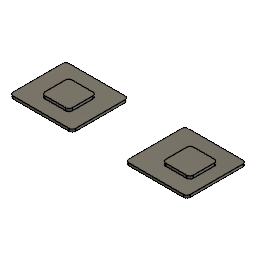
Joycon Drift Plugs v1 (Autodesk Fusion 360 design; units mm, degrees)
Autodesk Fusion 360 part; units mm, degrees
sketch "Sketch1" plane through (0, 0, 0) normal (0, 1, 0) x (1, 0, 0)
  line L0 (0, 0) -> (19, 0)
  line L1 (19, 0) -> (19, 17)
  line L2 (19, 17) -> (0, 17)
  line L3 (0, 17) -> (0, 0)
  line L4 (9.5, 0) -> (9.5, 12.3)
  line L5 (0, 8.5) -> (13.9, 8.5)
  line L6 (13.9, 12.3) -> (5.6, 12.3)
  line L7 (5.6, 12.3) -> (5.6, 4.1)
  line L8 (5.6, 4.1) -> (13.9, 4.1)
  line L9 (13.9, 4.1) -> (13.9, 12.3)
  dimension "d1" = 19
  dimension "d2" = 17
  dimension "d3" = 12.3
  dimension "d4" = 13.9
  dimension "d5" = 8.3
  dimension "d6" = 8.2
  constraint horizontal L0
  constraint vertical L1
  constraint horizontal L2
  constraint vertical L3
  constraint coincident L0.start L3.end
  constraint midpoint L0 L4.start
  constraint perpendicular L2 L4
  constraint midpoint L3 L5.start
  constraint perpendicular L4 L5
  constraint horizontal L6
  constraint vertical L7
  constraint horizontal L8
  constraint vertical L9
  measures "d1" distance of L0.start L0.end
  measures "d2" distance of L0.start L2.end
  measures "d3" distance of L4.start L4.end
  measures "d4" distance of L5.start L5.end
  measures "d5" distance of L6.start L6.end
  measures "d6" distance of L6.start L8.end
extrude "Extrude1" add sketch "Sketch1" along normal blind 1 makes body 1
extrude "Extrude2" add sketch "Sketch1" along normal blind 1.6 contours L4 L5 L7 L8 | L4 L5 L8 L9 | L4 L5 L6 L7 | L4 L5 L6 L9 bodies 1
extrude "Extrude3" cut 1 faces at (1.8667, 1, -9.7667) along direction (0, -1, 0) blind 0.2 on bodies 1 bodies 1
fillet "Fillet1" radius 1 4 edges at (5.6, 1.2, -4.1) (13.9, 1.2, -4.1) (13.9, 1.2, -12.3) (5.6, 1.2, -12.3) on bodies 1
fillet "Fillet2" radius 1 4 edges at (19, 0.4, -17) (0, 0.4, -17) (0, 0.4, 0) (19, 0.4, 0) on bodies 1
sketch "Sketch2" plane through (0, 0, 0) normal (0, 1, 0) x (1, 0, 0)
  line L0 (35, 0) -> (53.6, 0)
  line L1 (53.6, 0) -> (53.6, 18)
  line L2 (53.6, 18) -> (35, 18)
  line L3 (35, 18) -> (35, 0)
  line L4 (53.6, 9) -> (49.8, 9)
  line L5 (44.3, 18) -> (44.3, 13.1)
  line L6 (49.8, 13.1) -> (41.5, 13.1)
  line L7 (41.5, 13.1) -> (41.5, 4.7)
  line L8 (41.5, 4.7) -> (49.8, 4.7)
  line L9 (49.8, 4.7) -> (49.8, 13.1)
  dimension "d17" = 18.6
  dimension "d18" = 18
  dimension "d19" = 3.8
  dimension "d20" = 4.9
  dimension "d21" = 8.3
  dimension "d22" = 8.4
  constraint horizontal L0
  constraint vertical L1
  constraint horizontal L2
  constraint vertical L3
  constraint midpoint L1 L4.start
  constraint perpendicular L1 L4
  constraint midpoint L2 L5.start
  constraint perpendicular L2 L5
  constraint horizontal L6
  constraint vertical L7
  constraint horizontal L8
  constraint vertical L9
  measures "d17" distance of L0.start L0.end
  measures "d18" distance of L0.start L2.end
  measures "d19" distance of L4.start L4.end
  measures "d20" distance of L5.start L5.end
  measures "d21" distance of L6.start L6.end
  measures "d22" distance of L6.start L8.end
extrude "Extrude4" add sketch "Sketch2" along normal blind 0.8 separate body makes body 2
extrude "Extrude5" add sketch "Sketch2" along normal blind 1.6 contours L6 L7 L8 L9 bodies 2
fillet "Fillet3" radius 1 8 edges at (41.5, 1.2, -4.7) (35, 0.4, 0) (35, 0.4, -18) (49.8, 1.2, -13.1) (41.5, 1.2, -13.1) (53.6, 0.4, -18) (49.8, 1.2, -4.7) (53.6, 0.4, 0) on bodies 2
equation "d3 = 25.6 mm - 13.3 mm"
equation "d4 = 63.1 mm - 49.2 mm"
named bodies: "Joycon R", "Joycon L"
